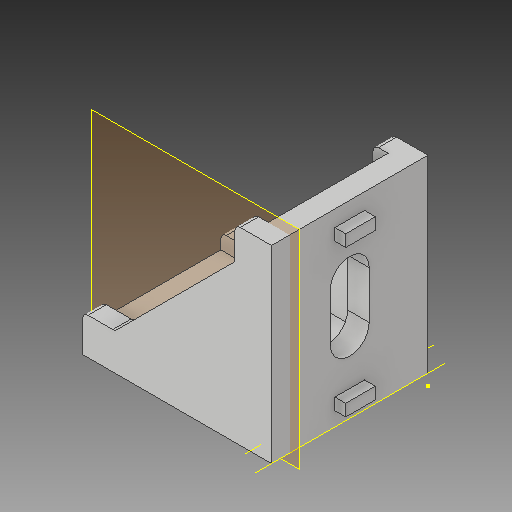
# Autodesk Inventor part: 30mm Bracket_CPY
Saved by Autodesk Inventor 2018 (Build 220112000, 112)
## iProperties
Created: 2016-07-11
Part Number: 30mm Bracket_CPY
Material: Generic
Document SubType Name: Modeling
Designer: User
Density: 1 g/cm^3
Appearance: Default
Author: joshm
Autodesk Inventor part; units mm, degrees
ref_plane "YZ Plane" through (0, 0, 0) normal (1, 0, 0) x (0, 1, 0)
ref_plane "XZ Plane" through (0, 0, 0) normal (0, 1, 0) x (-1, 0, 0)
ref_plane "XY Plane" through (0, 0, 0) normal (0, 0, 1) x (1, 0, 0)
sketch "Sketch1" plane through (0, 0, 0) normal (0, 0, 1) x (1, 0, 0)
  line L0 (0, 0) -> (0, 35)
  line L1 (0, 35) -> (-5.8, 35)
  line L2 (-6.8, 34) -> (-6.8, 29.4142)
  line L3 (0, 0) -> (-35, 0)
  line L4 (0, 0) -> (35, 0) construction
  line L5 (-35, 0) -> (-35, 5.8)
  line L6 (-34, 6.8) -> (-29.4142, 6.8)
  line L7 (-28.7071, 7.0929) -> (-7.0929, 28.7071)
  arc A0 (-5.8, 35) -> (-6.8, 34) centre (-5.8, 34) ccw
  arc A1 (-7.0929, 28.7071) -> (-6.8, 29.4142) centre (-7.8, 29.4142) ccw
  arc A2 (-29.4142, 6.8) -> (-28.7071, 7.0929) centre (-29.4142, 7.8) ccw
  arc A3 (-34, 6.8) -> (-35, 5.8) centre (-34, 5.8) ccw
  point P0 (-6.8, 35)
  point P1 (-6.8, 29)
  point P2 (-35, 6.8)
  point P3 (-29, 6.8)
  dimension "d0" = 35
  dimension "d1" = 6.8
  dimension "d2" = 90
  dimension "d3" = 6
  dimension "d4" = 35
  dimension "d5" = 180
  dimension "d6" = 6.8
  dimension "d7" = 6
  dimension "d8" = 90
  dimension "d9" = 1
  constraints: 16 end point, 8 point on circle, 8 point on line, 8 tangent, 4 centre point, 4 perpendicular, 3 equal radius, 2 horizontal, 1 collinear, 1 vertical
  measures "d0" distance of L0.start L0.end
  measures "d1" distance of L0.end point (-6.8, 35)
  measures "d2" angle of L1 L0
  measures "d3" distance of point (-6.8, 35) point (-6.8, 29)
  measures "d4" distance of L0.start L3.end
  measures "d5" angle of L3 L4
  measures "d6" distance of L3.end point (-35, 6.8)
  measures "d7" distance of point (-35, 6.8) point (-29, 6.8)
  measures "d8" angle of L5 L6
  measures "d9" radius of A0
extrude "Extrusion1" add sketch "Sketch1" along normal blind 29
ref_plane "Work Plane1" through (0, 0, 25.6) normal (0, 0, 1) x (1, 0, 0)
sketch "Sketch2" plane through (0, 0, 25.6) normal (0, 0, 1) x (1, 0, 0)
  line L0 (0, 0) -> (0, 35)
  line L1 (0, 35) -> (-5.8, 35)
  arc A0 (-5.8, 35) -> (-6.8, 34) centre (-5.8, 34) ccw
  line L2 (-6.8, 34) -> (-6.8, 29.4142)
  arc A1 (-7.0929, 28.7071) -> (-6.8, 29.4142) centre (-7.8, 29.4142) ccw
  line L3 (-7.0929, 28.7071) -> (-28.7071, 7.0929)
  arc A2 (-29.4142, 6.8) -> (-28.7071, 7.0929) centre (-29.4142, 7.8) ccw
  line L4 (-29.4142, 6.8) -> (-34, 6.8)
  arc A3 (-34, 6.8) -> (-35, 5.8) centre (-34, 5.8) ccw
  line L5 (-35, 5.8) -> (-35, 0)
  line L6 (-35, 0) -> (0, 0)
  line L7 (0, 0) -> (-4, 0)
  line L8 (-35, 0) -> (0, 0)
  line L9 (-4, 0) -> (-4, 35)
  line L10 (-4, 0) -> (-4, 4)
  line L11 (-4, 4) -> (-35, 4)
  line L12 (-35, 5.8) -> (-35, 0)
  line L13 (-4, 4) -> (-36.3789, 4)
  line L14 (-36.3789, 4) -> (-36.3789, 37.1754)
  line L15 (-36.3789, 37.1754) -> (-4, 37.1754)
  line L16 (-4, 37.1754) -> (-4, 4)
  dimension "d13" = 4
  constraints: 34 end point, 8 centre point, 8 point on circle, 3 point on line
  measures "d13" distance of L0.start L7.end
extrude "Extrusion2" cut sketch "Sketch2" against normal blind 22.2 contours L9 L11 L5 A3 L4 A2 L3 A1 L2 A0 L1
sketch "Sketch3" plane through (-35, 4, 25.6) normal (0, 1, 0) x (1, 0, 0)
  line L0 (0, 0) -> (0, 22.2) projected
  line L1 (0, 11.1) -> (9, 11.1)
  line L2 (9, 11.1) -> (12.6, 11.1)
  arc A0 (12.6, 14.7) -> (12.6, 7.5) centre (12.6, 11.1) ccw
  line L3 (17.8, 11.1) -> (25, 11.1)
  line L4 (25, 11.1) -> (21.4, 11.1)
  arc A1 (21.4, 7.5) -> (21.4, 14.7) centre (21.4, 11.1) ccw
  line L5 (12.6, 14.7) -> (21.4, 14.7)
  line L6 (12.6, 7.5) -> (21.4, 7.5)
  point P0 (35, 25.6)
  dimension "d16" = 9
  dimension "d17" = 3.6
  dimension "d18" = 16
  dimension "d19" = 3.6
  constraints: 12 end point, 6 point on circle, 2 centre point, 2 coincident, 2 midpoint, 2 point on line, 2 tangent, 1 horizontal
  measures "d16" distance of L1.start L1.end
  measures "d17" distance of L1.end L2.end
  measures "d18" distance of L1.end L3.end
  measures "d19" distance of L3.end L4.end
extrude "Extrusion3" cut sketch "Sketch3" against normal blind 22.2
fillet "Fillet1" radius 1 1 edges at (-4, 4, 14.5)
sketch "Sketch4" plane through (0, 0, 0) normal (0, 0, -1) x (-1, 0, 0)
  line L0 (5, 4) -> (35, 4) projected
  line L1 (4, 35) -> (4, 5) projected
  line L2 (0, 0) -> (0, 2)
  line L3 (0, 0) -> (0, 35) projected
  line L4 (0, 2) -> (0, 0)
  line L5 (0, 2) -> (2, 2)
  dimension "d23" = 2
  dimension "d24" = 2
  dimension "d25" = 2
  constraints: 6 end point, 1 collinear, 1 horizontal, 1 point on line
  measures "d23" distance of L2.start L2.end
  measures "d24" distance of L2.end L2.start
  measures "d25" distance of L2.end L5.end
pattern_circular "Circular Pattern1" count 2 over 270 about axis through (-2, 2, 0) along (0, 0, 1) of "Extrusion3"
sketch "Sketch5" plane through (-35, 0, 0) normal (0, -1, 0) x (1, 0, 0)
  line L0 (0, 25.6) -> (0, 3.4) projected
  line L1 (0, 14.5) -> (3, 14.5)
  line L2 (0, 14.5) -> (3, 14.5) construction
  line L3 (3, 14.5) -> (3, 11.75)
  line L4 (3, 11.75) -> (3, 17.25)
  line L5 (3, 17.25) -> (5.2, 17.25)
  line L6 (5.2, 17.25) -> (5.2, 11.75)
  line L7 (5.2, 11.75) -> (3, 11.75)
  line L8 (35, 0) -> (35, 29) projected
  line L9 (35, 14.5) -> (32.4, 14.5)
  line L10 (32.4, 14.5) -> (32.4, 11.75)
  line L11 (32.4, 11.75) -> (30.2, 11.75)
  line L12 (30.2, 11.75) -> (30.2, 17.25)
  line L13 (30.2, 17.25) -> (32.4, 17.25)
  line L14 (32.4, 17.25) -> (32.4, 11.75)
  dimension "d29" = 3
  dimension "d30" = 0
  dimension "d31" = 2.75
  dimension "d32" = 5.5
  dimension "d33" = 2.2
  dimension "d34" = 2.6
  dimension "d35" = 2.75
  dimension "d36" = 2.2
  dimension "d37" = 5.5
  constraints: 26 end point, 6 perpendicular, 4 horizontal, 2 midpoint, 2 parallel, 1 collinear, 1 point on line
  measures "d29" distance of L1.start L1.end
  measures "d30" distance between parallel lines of L1 L2
  measures "d31" distance of L1.end L3.end
  measures "d32" distance of L3.end L4.end
  measures "d33" distance of L4.end L5.end
  measures "d34" distance of L9.start L9.end
  measures "d35" distance of L9.end L10.end
  measures "d36" distance of L12.end L13.end
  measures "d37" distance of L11.end L12.end
extrude "Extrusion4" add sketch "Sketch5" along normal blind 2
sketch "Sketch7" plane through (-35, -2, 0) normal (0, -1, 0) x (1, 0, 0)
  point P0 (35, 0)
sketch "Sketch9" plane through (0, 0, 0) normal (1, 0, 0) x (0, 0, -1)
  line L0 (-10.9, 22.4) -> (-10.9, 13.6) projected
  arc A0 (-18.1, 13.6) -> (-10.9, 13.6) centre (-14.5, 13.6) ccw projected
  line L1 (-18.1, 13.6) -> (-18.1, 22.4) projected
  arc A1 (-10.9, 22.4) -> (-18.1, 22.4) centre (-14.5, 22.4) ccw projected
  line L2 (0, 0) -> (0, 35) projected
  line L3 (0, 35) -> (-29, 35) projected
  line L4 (-29, 0) -> (-29, 35) projected
  line L5 (0, 0) -> (-29, 0) projected
  line L6 (-11.75, 32) -> (-11.75, 29.8) projected
  line L7 (-11.75, 32) -> (-17.25, 32)
  line L8 (-17.25, 32) -> (-17.25, 29.8)
  line L9 (-17.25, 29.8) -> (-11.75, 29.8)
  line L10 (-11.75, 29.8) -> (-11.75, 32)
  line L11 (-11.75, 2.6) -> (-17.25, 2.6) projected
  line L12 (-11.75, 4.8) -> (-17.25, 4.8)
  line L13 (-17.25, 4.8) -> (-17.25, 2.6)
  line L14 (-17.25, 2.6) -> (-11.75, 2.6)
  line L15 (-11.75, 2.6) -> (-11.75, 4.8)
  constraints: 16 end point, 4 parallel, 2 horizontal, 2 perpendicular
extrude "Extrusion5" add sketch "Sketch9" along normal blind 2 contours L6 L9 L8 L7 | L11 L13 L12 L15
sketch "Sketch10" plane through (-4, 35, 3.4) normal (-1, 0, 0) x (0, 0, 1)
  point P0 (-3.4, -35)
body "Solid1"
